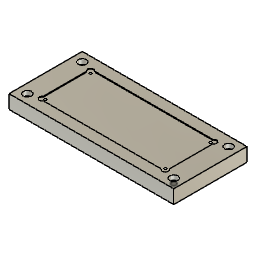
CAD_File 2 (Autodesk Fusion 360 design; units mm, degrees)
Autodesk Fusion 360 part; units mm, degrees
sketch "Sketch14" plane through (0, 0, 0) normal (0, 0, 1) x (1, 0, 0)
  line L0 (-112.5, -50) -> (112.5, -50)
  line L1 (112.5, -50) -> (112.5, 50)
  line L2 (112.5, 50) -> (-112.5, 50)
  line L3 (-112.5, 50) -> (-112.5, -50)
  line L4 (-112.5, -50) -> (112.5, 50) construction
  line L5 (112.5, -50) -> (-112.5, 50) construction
  dimension "d46" = 225
  dimension "d47" = 100
  constraint horizontal L0
  constraint perpendicular L0 L1
  constraint parallel L0 L2
  constraint parallel L1 L3
  constraint coincident L4 origin
  constraint coincident L5 origin
  measures "d46" distance of L1.end L2.end
  measures "d47" distance of L0.end L1.end
extrude "Extrude10" add sketch "Sketch14" along normal blind 18.7
sketch "Sketch15" plane through (0, 0, 18.7) normal (0, 0, 1) x (-1, 0, 0)
  line L0 (112.5, -50) -> (112.5, 50)
  line L1 (112.5, 50) -> (-112.5, 50)
  line L2 (-112.5, 50) -> (-112.5, -50)
  line L3 (-112.5, -50) -> (112.5, -50)
  line L4 (80.5859, 35.05) -> (-80.5859, 35.05)
  line L5 (-86.05, 29.5859) -> (-86.05, -29.5859)
  line L6 (-80.5859, -35.05) -> (80.5859, -35.05)
  line L7 (86.05, -29.5859) -> (86.05, 29.5859)
  line L8 (86.05, 35.05) -> (-86.05, -35.05) construction
  line L9 (-86.05, 35.05) -> (86.05, -35.05) construction
  line L10 (0, -40) -> (0, 40) construction
  line L11 (90, 0) -> (-90, 0) construction
  arc A0 (80.5859, -35.05) -> (86.05, -29.5859) centre (84.05, -33.05) ccw
  arc A1 (-86.05, -29.5859) -> (-80.5859, -35.05) centre (-84.05, -33.05) ccw
  arc A2 (-80.5859, 35.05) -> (-86.05, 29.5859) centre (-84.05, 33.05) ccw
  arc A3 (86.05, 29.5859) -> (80.5859, 35.05) centre (84.05, 33.05) ccw
  dimension "d50" = 172.1
  dimension "d51" = 70.1
  dimension "d89" = 8
  dimension "d90" = 2
  dimension "d91" = 2
  constraint horizontal L4
  constraint perpendicular L4 L5
  constraint parallel L4 L6
  constraint parallel L5 L7
  constraint coincident L8 origin
  constraint coincident L9 origin
  constraint vertical L10
  constraint perpendicular L7 L11
  constraint symmetric L10 A0 A1
  constraint symmetric L11 A0 A3
  constraint symmetric L11 A1 A2
  measures "d50" distance of L8.end L9.end
  measures "d51" distance of L9.start L8.end
  measures "d89" diameter of A0
  measures "d90" distance of L6 A0.centre
  measures "d91" distance of L7 A0.centre
extrude "Extrude11" cut sketch "Sketch15" against normal blind 1 contours L4 L5 L6 L7 A0 A1 A2 A3
sketch "Sketch16" plane through (0, 0, 18.7) normal (0, 0, 1) x (-1, 0, 0)
  line L0 (86.1, -35.1) -> (86.1, 35.1)
  line L1 (86.1, 35.1) -> (-86.1, 35.1)
  line L2 (-86.1, 35.1) -> (-86.1, -35.1)
  line L3 (-86.1, -35.1) -> (86.1, -35.1)
  circle A0 centre (100, -37.5) radius 5.5
  circle A1 centre (100, 37.5) radius 5.5
  circle A2 centre (-100, -37.5) radius 5.5
  circle A3 centre (-100, 37.5) radius 5.5
  line L4 (112.5, -50) -> (112.5, 50)
  line L5 (-112.5, -50) -> (112.5, -50)
  line L6 (112.5, 50) -> (-112.5, 50)
  line L7 (-112.5, 50) -> (-112.5, -50)
  line L8 (-80.5859, 35.05) -> (80.5859, 35.05)
  line L9 (86.05, 29.5859) -> (86.05, -29.5859)
  line L10 (80.5859, -35.05) -> (-80.5859, -35.05)
  line L11 (-86.05, -29.5859) -> (-86.05, 29.5859)
  line L12 (112.5, -50) -> (112.5, 50)
  line L13 (112.5, 50) -> (-112.5, 50)
  line L14 (-112.5, 50) -> (-112.5, -50)
  line L15 (-112.5, -50) -> (112.5, -50)
  arc A4 (86.05, 29.5859) -> (80.5859, 35.05) centre (84.05, 33.05) ccw
  arc A5 (80.5859, -35.05) -> (86.05, -29.5859) centre (84.05, -33.05) ccw
  arc A6 (-86.05, -29.5859) -> (-80.5859, -35.05) centre (-84.05, -33.05) ccw
  arc A7 (-80.5859, 35.05) -> (-86.05, 29.5859) centre (-84.05, 33.05) ccw
  dimension "d54" = 11
  dimension "d55" = 11
  dimension "d56" = 11
  dimension "d57" = 11
  dimension "d58" = 12.5
  dimension "d59" = 12.5
  dimension "d60" = 12.5
  dimension "d61" = 12.5
  dimension "d62" = 12.5
  dimension "d63" = 12.5
  dimension "d64" = 12.5
  dimension "d65" = 12.5
  measures "d54" diameter of A0
  measures "d55" diameter of A1
  measures "d56" diameter of A2
  measures "d57" diameter of A3
  measures "d58" distance of A0.centre L4
  measures "d59" distance of A0.centre L5
  measures "d60" distance of A1.centre L6
  measures "d61" distance of A1.centre L4
  measures "d62" distance of A2.centre L5
  measures "d63" distance of A2.centre L7
  measures "d64" distance of A3.centre L7
  measures "d65" distance of A3.centre L6
extrude "Extrude12" cut sketch "Sketch16" against normal blind 6.5 contours A0 | A1 | A2 | A3
sketch "Sketch17" plane through (0, 0, 12.2) normal (0, 0, 1) x (-1, 0, 0)
  circle A0 centre (100, -37.5) radius 5.5
  circle A1 centre (100, -37.5) radius 3
  dimension "d68" = 6
  constraint concentric A0 A1
  measures "d68" diameter of A1
sketch "Sketch18" plane through (0, 0, 12.2) normal (0, 0, 1) x (-1, 0, 0)
  circle A0 centre (-100, -37.5) radius 5.5
  circle A1 centre (-100, -37.5) radius 3
  dimension "d69" = 6
  constraint concentric A0 A1
  measures "d69" diameter of A1
sketch "Sketch19" plane through (0, 0, 12.2) normal (0, 0, 1) x (-1, 0, 0)
  circle A0 centre (-100, 37.5) radius 5.5
  circle A1 centre (-100, 37.5) radius 3
  dimension "d70" = 6
  constraint concentric A0 A1
  measures "d70" diameter of A1
sketch "Sketch20" plane through (0, 0, 12.2) normal (0, 0, 1) x (-1, 0, 0)
  circle A0 centre (100, 37.5) radius 5.5
  circle A1 centre (100, 37.5) radius 3
  dimension "d71" = 6
  constraint concentric A0 A1
  measures "d71" diameter of A1
extrude "Extrude13" cut sketch "Sketch18" sketch "Sketch17" sketch "Sketch20" sketch "Sketch19" along normal up to surface contours A1 of sketch 2 contours A1 of sketch 3 contours A1 of sketch 4 contours A1 end surface through (0, 0, 0) normal (0, 0, -1) offset 0
sketch "Sketch21" plane through (0, 0, 17.7) normal (0, 0, 1) x (-1, 0, 0)
  line L0 (86.05, -29.5859) -> (86.05, 29.5859)
  line L1 (80.5859, 35.05) -> (-80.5859, 35.05)
  line L2 (-86.05, 29.5859) -> (-86.05, -29.5859)
  line L3 (-80.5859, -35.05) -> (80.5859, -35.05)
  circle A0 centre (81.95, -30.95) radius 2
  circle A1 centre (-81.95, -30.95) radius 2
  circle A2 centre (-81.95, 30.95) radius 2
  circle A3 centre (81.95, 30.95) radius 2
  arc A4 (86.05, 29.5859) -> (80.5859, 35.05) centre (84.05, 33.05) ccw
  arc A5 (-80.5859, 35.05) -> (-86.05, 29.5859) centre (-84.05, 33.05) ccw
  arc A6 (-86.05, -29.5859) -> (-80.5859, -35.05) centre (-84.05, -33.05) ccw
  arc A7 (80.5859, -35.05) -> (86.05, -29.5859) centre (84.05, -33.05) ccw
  dimension "d74" = 4
  dimension "d75" = 4
  dimension "d76" = 4
  dimension "d77" = 4
  dimension "d78" = 4.1
  dimension "d79" = 4.1
  dimension "d80" = 4.1
  dimension "d81" = 4.1
  dimension "d82" = 4.1
  dimension "d83" = 4.1
  dimension "d84" = 4.1
  dimension "d85" = 4.1
  measures "d74" diameter of A0
  measures "d75" diameter of A1
  measures "d76" diameter of A2
  measures "d77" diameter of A3
  measures "d78" distance of L0 A0.centre
  measures "d79" distance of L3 A0.centre
  measures "d80" distance of L1 A3.centre
  measures "d81" distance of L0 A3.centre
  measures "d82" distance of L3 A1.centre
  measures "d83" distance of L2 A1.centre
  measures "d84" distance of L1 A2.centre
  measures "d85" distance of L2 A2.centre
extrude "Extrude14" cut sketch "Sketch21" against normal blind 20 contours A0 | A1 | A2 | A3
thread "Thread1" "ISO Metric profile 4.0 M4x0.7 6H" major diameter 4.1095 minor diameter 3.332 pitch 0.7 angle 60 resizes the face on face at (-82.1987, 32.9345, 11.8) on face at (-83.3465, -32.3817, 11.8) on face at (80.5535, -32.3817, 11.8) on face at (80.5535, 29.5183, 11.8)
sketch "Sketch4" plane through (0, 0, 2) normal (0, 0, 1) x (-1, 0, 0)
  circle A0 centre (-75, -25) radius 5.5
  circle A1 centre (-75, -25) radius 3.1
  dimension "d20" = 6.2
  constraint concentric A0 A1
  measures "d20" diameter of A1
sketch "Sketch5" plane through (0, 0, 2) normal (0, 0, 1) x (-1, 0, 0)
  circle A0 centre (-75, 25) radius 5.5
  circle A1 centre (-75, 25) radius 3.1
  dimension "d21" = 6.2
  constraint concentric A0 A1
  measures "d21" diameter of A1
sketch "Sketch6" plane through (0, 0, 2) normal (0, 0, 1) x (-1, 0, 0)
  circle A0 centre (75, 25) radius 5.5
  circle A1 centre (75, 25) radius 3.1
  dimension "d22" = 6.2
  constraint concentric A0 A1
  measures "d22" diameter of A1
